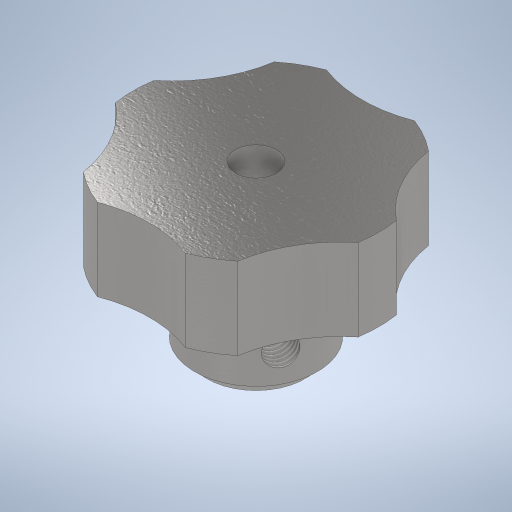
# Autodesk Inventor part: bolt
Saved by Autodesk Inventor 2024 (Build 280153000, 153)
## iProperties
Created: 2024-02-02
Part Number: bolt
Material: Stahl, galvanisiert
Document SubType Name: Modeling
Designer: ffogue
Density: 7.85 g/cm^3
Appearance: Galvanisiert
Author: ffogue
Autodesk Inventor part; units mm, degrees
ref_plane "YZ Plane" through (0, 0, 0) normal (1, 0, 0) x (0, 1, 0)
ref_plane "XZ Plane" through (0, 0, 0) normal (0, 1, 0) x (-1, 0, 0)
sketch "Skizze1" plane through (0, 0, 0) normal (0, 0, 1) x (1, 0, 0)
  circle A0 centre (0, 0) radius 15
  line L0 (0, 15) -> (0, -15) construction
  arc A1 (-5.3852, 14) -> (5.3852, 14) centre (0, 28) ccw
  point P0 (0, 0)
  point P1 (0, 13)
  dimension "d0" = 30
  dimension "d1" = 15
  dimension "d2" = 13
  constraints: 7 point on circle, 2 centre point, 2 coincident, 2 end point, 1 midpoint, 1 symmetric about line, 1 vertical, 1 vertical alignment
  measures "d0" diameter of A0
  measures "d1" radius of A1
  measures "d2" distance of point (0, 0) point (0, 13)
extrude "Extrusion1" add sketch "Skizze1" along normal blind 10
extrude "Extrusion2" cut sketch "Skizze1" along normal blind 10 contours A1 A0 picked at (0.6105, 13.7041)
pattern_circular "Runde Anordnung1" count 6 over 360 about axis through (0, 0, 0) along (0, 0, 1) of "Extrusion2"
sketch "Skizze2" plane through (0, 0, 0) normal (0, 0, -1) x (-1, 0, 0)
  circle A0 centre (0, 0) radius 7.5
  dimension "d10" = 15
  constraints: 1 centre point, 1 coincident
  measures "d10" diameter of A0
extrude "Extrusion3" add sketch "Skizze2" along normal blind 10
chamfer "Fasen1" distance 1.5 angle 45 1 edges at (7.5, 0, -10)
sketch "Skizze3" plane through (0, 0, 10) normal (0, 0, 1) x (1, 0, 0)
  circle A0 centre (0, 0) radius 2.5
  dimension "d16" = 5
  constraints: 1 centre point, 1 coincident
  measures "d16" diameter of A0
extrude "Extrusion4" cut sketch "Skizze3" against normal up to surface (20 mm away)
ref_plane "Arbeitsebene2" through (-5.3852, -14, 0) normal (0.8825, -0.4703, 0) x (0.4703, 0.8825, 0)
sketch "Skizze5" plane through (-5.3852, -14, 0) normal (0.8825, -0.4703, 0) x (0.4703, 0.8825, 0)
  circle A0 centre (14.8877, -5) radius 1.75
  point P0 (14.8877, 0)
  dimension "d21" = 3.5
  dimension "d22" = 5
  constraints: 1 centre point, 1 vertical alignment
  measures "d21" diameter of A0
  measures "d22" distance of point (14.888, 0) A0.centre
extrude "Extrusion5" cut sketch "Skizze5" along normal through all both and the other way through all
thread "Gewinde2" size "M3.5x0.6" class "6H" standard "ANSI Metric M Profile" length 25
thread "Gewinde3" size "M3.5x0.6" class "6H" standard "ANSI Metric M Profile" length 25
